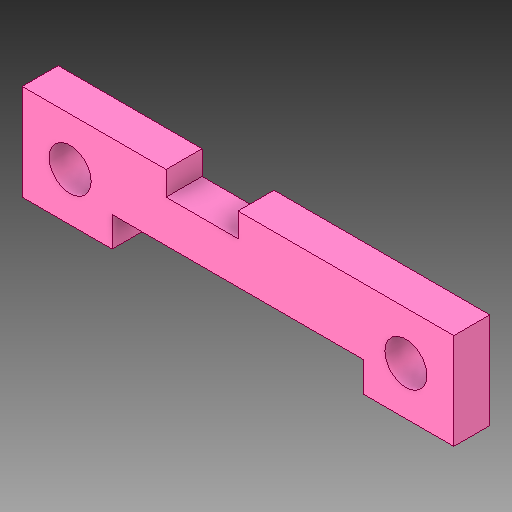
# Autodesk Inventor part: solar_board_holder
Saved by Autodesk Inventor 2018 (Build 220112000, 112)
## iProperties
Created: 2019-04-03
Part Number: solar_board_holder
Material: Generic
Document SubType Name: Modeling
Designer: ZEUSLAP
Density: 1 g/cm^3
Appearance: Default
Mass: 0.594773 g
Surface Area: 7.67489 cm^2
Volume: 0.594773 cm^3
Author: ZEUSLAP
## iProperties of the stored document solar_board_holder_3DPrint.ipt
Created: 2019-04-13
Part Number: solar_board_holder_3DPrint
Material: Generic
Document SubType Name: Modeling
Designer: ZEUSLAP
Density: 1 g/cm^3
Appearance: Default
Author: ZEUSLAP
Autodesk Inventor part; units mm, degrees
ref_plane "YZ Plane" through (0, 0, 0) normal (1, 0, 0) x (0, 1, 0)
ref_plane "XZ Plane" through (0, 0, 0) normal (0, 1, 0) x (-1, 0, 0)
ref_plane "XY Plane" through (0, 0, 0) normal (0, 0, 1) x (1, 0, 0)
sketch "Sketch" plane through (0, 0, 0) normal (0, 0, 1) x (1, 0, 0)
  line L0 (-18, -4) -> (-18, 4)
  circle A0 centre (-14, 0) radius 1.75
  circle A1 centre (14, 0) radius 1.75
  line L1 (-10.5, -1.5) -> (-10.5, -4)
  line L2 (10.5, -1.5) -> (10.5, -4)
  line L3 (-18, -4) -> (-10.5, -4)
  line L4 (10.5, -4) -> (18, -4)
  line L5 (-6, 4) -> (-6, 2)
  line L6 (-6, 2) -> (0, 2)
  line L7 (0, 2) -> (0, 4)
  line L8 (0, 4) -> (11.6122, 4)
  line L9 (0, 4) -> (18, 4)
  line L10 (18, 4) -> (18, -4)
  line L11 (-10.5, -1.5) -> (10.5, -1.5)
  line L12 (-6, 4) -> (-18, 4)
  line L13 (0, 15.3827) -> (0, -14.6173) construction
  point P0 (0, 0)
  point P1 (18, 0)
  dimension "d18" = 3.5
  dimension "d34" = 6
  dimension "d35" = 21
  dimension "d36" = 2.5
  dimension "d39" = 36
  dimension "d41" = 8
  dimension "d45" = 12
  dimension "d49" = 14
  dimension "d50" = 28
  dimension "d51" = 2
  constraints: 28 end point, 6 perpendicular, 4 equal length, 3 horizontal, 2 centre point, 2 vertical, 1 equal radius, 1 horizontal alignment, 1 midpoint, 1 point on line, 2 other
  measures "d18" diameter of A0
  measures "d34" distance between parallel lines of L7 L5
  measures "d35" distance between parallel lines of L2 L1
  measures "d36" distance of L1.start L1.end
  measures "d39" distance between parallel lines of L10 L0
  measures "d41" distance of L0.start L0.end
  measures "d45" distance of L5.start L0.end
  measures "d49" distance of point (0, 0) A0.centre
  measures "d50" distance of A1.centre A0.centre
  measures "d51" distance of L6.end L7.end
extrude "holder" add sketch "Sketch" along normal blind 3
sketch "Sketch3" plane through (0, 0, 0) normal (0, 0, -1) x (-1, 0, 0)
  line L0 (10.5, -1.5) -> (-10.5, -1.5) projected
  line L1 (-9, 0.5) -> (9, 0.5)
  line L2 (9, 0.5) -> (9, -1.5)
  line L3 (9, -1.5) -> (-9, -1.5)
  line L4 (-9, -1.5) -> (-9, 0.5)
  point P0 (0, 0)
  point P1 (0, -1.5)
  dimension "d52" = 2
  dimension "d53" = 18
  constraints: 8 end point, 2 parallel, 1 collinear, 1 horizontal, 1 midpoint, 1 perpendicular, 1 vertical alignment
  measures "d52" distance of L1.end L2.end
  measures "d53" distance of L1.start L1.end
extrude "cutout for connector legs" cut sketch "Sketch3" against normal blind 0.5
body "Solid4"
